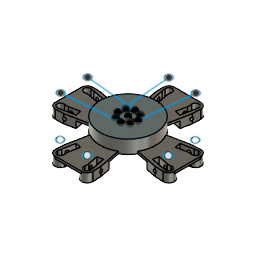
UpperMoulding_v12 (Autodesk Fusion 360 design; units mm, degrees)
Autodesk Fusion 360 part; units mm, degrees
sketch "Sketch3" plane through (0, 0, 0) normal (0, 0, 1) x (1, 0, 0)
  line L0 (-12, 0) -> (12, 0)
  line L1 (0, 0) -> (0, 60) construction
  line L2 (-12, 0) -> (0, 60) construction
  line L3 (0, 60) -> (12, 0) construction
  line L4 (-14.4515, 0.4903) -> (-9.5485, -0.4903)
  line L5 (-14.4515, 0.4903) -> (-9.5485, -0.4903)
  line L6 (-9.5485, -0.4903) -> (-7.5874, 9.3155)
  line L7 (-7.5874, 9.3155) -> (-12.4903, 10.2961)
  line L8 (-12.4903, 10.2961) -> (-14.4515, 0.4903)
  line L9 (-13.4709, 5.3932) -> (-16.4126, 5.9815) construction
  line L10 (-12, -3.0594) -> (12, -3.0594) construction
  circle A0 centre (-12, -3.0594) radius 3
  line L11 (0, 0) -> (0, -3.0594) construction
  line L12 (-14.4515, 0.4903) -> (-14.9594, -2.5678)
  line L13 (-9.5485, -0.4903) -> (-9.0891, -2.3339)
  line L14 (-8.568, 4.4126) -> (-5.6262, 3.8243) construction
  line L15 (-16.1184, 7.4524) -> (-16.7068, 4.5107)
  line L16 (-5.3321, 5.2951) -> (-5.9204, 2.3534)
  line L17 (-16.1184, 7.4524) -> (-13.1767, 6.8641) construction
  line L18 (-16.7068, 4.5107) -> (-13.765, 3.9223) construction
  line L19 (-5.9204, 2.3534) -> (-8.8621, 2.9417) construction
  line L20 (-5.3321, 5.2951) -> (-8.2738, 5.8835) construction
  circle A1 centre (-12, -3.0594) radius 5
  line L21 (-16.7068, 4.5107) -> (-16.9962, -2.8634)
  line L22 (-5.9204, 2.3534) -> (-7.0825, -3.964)
  line L23 (-10.0388, 9.8058) -> (-9.4505, 12.7475)
  line L24 (-16.1184, 7.4524) -> (-14.8437, 13.8262)
  line L25 (-14.8437, 13.8262) -> (-9.4505, 12.7475)
  line L26 (-5.3321, 5.2951) -> (-4.0573, 11.6689)
  line L27 (-4.0573, 11.6689) -> (-9.4505, 12.7475)
  line L28 (9.5485, -0.4903) -> (14.4515, 0.4903)
  line L29 (9.5485, -0.4903) -> (14.4515, 0.4903)
  line L30 (14.4515, 0.4903) -> (12.4903, 10.2961)
  line L31 (12.4903, 10.2961) -> (7.5874, 9.3155)
  line L32 (7.5874, 9.3155) -> (9.5485, -0.4903)
  circle A2 centre (12, -3.0594) radius 3
  line L33 (9.5485, -0.4903) -> (9.0891, -2.3339)
  line L34 (14.4515, 0.4903) -> (14.9594, -2.5678)
  circle A3 centre (12, -3.0594) radius 5
  line L35 (13.4709, 5.3932) -> (16.4126, 5.9815) construction
  line L36 (8.568, 4.4126) -> (5.6262, 3.8243) construction
  line L37 (16.1184, 7.4524) -> (16.7068, 4.5107)
  line L38 (5.3321, 5.2951) -> (5.9204, 2.3534)
  line L39 (5.9204, 2.3534) -> (7.0825, -3.964)
  line L40 (16.7068, 4.5107) -> (16.9962, -2.8634)
  line L41 (10.0388, 9.8058) -> (9.4505, 12.7475) construction
  line L42 (9.4505, 12.7475) -> (14.8437, 13.8262)
  line L43 (14.8437, 13.8262) -> (16.1184, 7.4524)
  line L44 (9.4505, 12.7475) -> (4.0573, 11.6689)
  line L45 (4.0573, 11.6689) -> (5.3321, 5.2951)
  line L46 (-4.0573, 11.6689) -> (4.0573, 11.6689)
  line L47 (-12, -8.0594) -> (12, -8.0594)
  point P0 (0, -3.0594)
  dimension "d11" = 24
  dimension "d12" = 60
  dimension "d13" = 5
  dimension "d14" = 10
  dimension "d15" = 3
  dimension "d16" = 24
  dimension "d17" = 6
  dimension "d18" = 3
  dimension "d19" = 3
  dimension "d20" = 3
  dimension "d21" = 2
  dimension "d22" = 3
  dimension "d23" = 5
  dimension "d24" = 10
  dimension "d25" = 6
  dimension "d26" = 2
  dimension "d27" = 3
  dimension "d28" = 3
  dimension "d29" = 3
  dimension "d30" = 3
  dimension "d31" = 3
  constraint midpoint L0 L1.start
  constraint coincident L1.start L11.start
  constraint horizontal L0
  constraint vertical L1
  constraint midpoint L0.start L4
  constraint perpendicular L2 L4
  constraint perpendicular L5 L6
  constraint parallel L5 L7
  constraint parallel L6 L8
  constraint midpoint L8 L9.start
  constraint perpendicular L8 L9
  constraint midpoint L10 P0
  constraint perpendicular L1 L10
  constraint coincident L10.start A0.centre
  constraint coincident P0 L11.end
  constraint perpendicular L10 L11
  constraint tangent L5 A0
  constraint coincident A0 L12.end
  constraint tangent A0 L12
  constraint coincident A0 L13.end
  constraint tangent A0 L13
  constraint midpoint L6 L14.start
  constraint perpendicular L6 L14
  constraint midpoint L9.end L15
  constraint perpendicular L9 L15
  constraint midpoint L14.end L16
  constraint perpendicular L14 L16
  constraint coincident L8 L17.end
  constraint perpendicular L8 L17
  constraint coincident L8 L18.end
  constraint perpendicular L8 L18
  constraint coincident L6 L19.end
  constraint perpendicular L6 L19
  constraint coincident L6 L20.end
  constraint perpendicular L6 L20
  constraint concentric A0 A1
  constraint coincident A1 L21.end
  constraint tangent A1 L21
  constraint coincident A1 L22.end
  constraint tangent A1 L22
  constraint midpoint L7 L23.start
  constraint perpendicular L7 L23
  constraint perpendicular L17 L24
  constraint perpendicular L20 L26
  constraint perpendicular L24 L25
  constraint perpendicular L26 L27
  constraint midpoint L0.end L28
  constraint perpendicular L3 L28
  constraint perpendicular L29 L30
  constraint parallel L29 L31
  constraint parallel L30 L32
  constraint coincident L10.end A2.centre
  constraint coincident A2 L33.end
  constraint tangent A2 L33
  constraint coincident A2 L34.end
  constraint tangent A2 L34
  constraint concentric A2 A3
  constraint midpoint L30 L35.start
  constraint perpendicular L30 L35
  constraint midpoint L32 L36.start
  constraint perpendicular L32 L36
  constraint midpoint L35.end L37
  constraint perpendicular L35 L37
  constraint midpoint L36.end L38
  constraint perpendicular L36 L38
  constraint coincident A3 L39.end
  constraint tangent A3 L39
  constraint coincident A3 L40.end
  constraint tangent A3 L40
  constraint midpoint L31 L41.start
  constraint perpendicular L31 L41
  constraint perpendicular L41 L42
  constraint perpendicular L41 L44
  constraint perpendicular L44 L45
  constraint perpendicular L42 L43
  constraint coincident A1 L47.start
  constraint coincident A3 L47.end
  constraint tangent A1 L47
  constraint tangent A3 L47
  measures "d11" distance of L0.start L0.end
  measures "d12" distance of L1.start L1.end
  measures "d13" distance of L4.start L4.end
  measures "d14" distance of L4.start L7.end
  measures "d15" distance of L9.start L9.end
  measures "d16" distance of L10.start L10.end
  measures "d17" diameter of A0
  measures "d18" distance of L14.start L14.end
  measures "d19" distance of L15.start L15.end
  measures "d20" distance of L16.start L16.end
  measures "d21" distance of A0 A1
  measures "d22" distance of L23.start L23.end
  measures "d23" distance of L28.start L28.end
  measures "d24" distance of L28.start L31.end
  measures "d25" diameter of A2
  measures "d26" distance of A2 A3
  measures "d27" distance of L35.start L35.end
  measures "d28" distance of L36.start L36.end
  measures "d29" distance of L37.start L37.end
  measures "d30" distance of L38.start L38.end
  measures "d31" distance of L41.start L41.end
extrude "Extrude4" add sketch "Sketch3" along normal blind 8 contours L0 L6 A1 | L0 L6 L8 A0 L12 L13 A1 | L0 L6 L7 L16 A1 L22 L23 L26 L27 | L0 A1 L22 | L7 L8 L15 A1 L21 L23 L24 L25 | L0 L30 L31 L32 A3 L37 L38 L39 L40 L42 L43 L44 L45 | L0 A3 L39 | L0 L32 A3 | L0 L30 L32 A2 L33 L34 A3 makes body 1 at (-10.4638, 11.9304, 0) makes body 2 at (10.4638, 11.9304, 0)
sketch "Sketch4" plane through (-16.9317, 3.3863, 0) normal (-0.980581, 0.196116, 0) x (-0.196116, -0.980581, 0)
  line L0 (-10.6466, 0) -> (-1.1466, 0)
  line L1 (-1.1466, 0) -> (-1.1466, 8)
  line L2 (-1.1466, 8) -> (-10.6466, 8)
  line L3 (-10.6466, 8) -> (-10.6466, 0)
  line L4 (-1.1466, 4) -> (-1.6466, 4) construction
  circle A0 centre (-1.6466, 4) radius 1.5
  dimension "d34" = 3
  dimension "d41" = 0.5
  constraint midpoint L1 L4.start
  constraint perpendicular L1 L4
  constraint coincident L4.end A0.centre
  measures "d34" diameter of A0
  measures "d41" distance of L4.start L4.end
extrude "Extrude5" cut sketch "Sketch4" against normal blind 10 contours L1 A0 | L1 A0 bodies 1
sketch "Sketch5" plane through (16.9317, 3.3863, 0) normal (0.980581, 0.196116, 0) x (-0.196116, 0.980581, 0)
  line L0 (1.1466, 0) -> (10.6466, 0)
  line L1 (10.6466, 0) -> (10.6466, 8)
  line L2 (10.6466, 8) -> (1.1466, 8)
  line L3 (1.1466, 8) -> (1.1466, 0)
  line L4 (1.1466, 4) -> (1.6466, 4) construction
  circle A0 centre (1.6466, 4) radius 1.5
  dimension "d37" = 0.5
  dimension "d38" = 3
  constraint midpoint L3 L4.start
  constraint perpendicular L3 L4
  constraint coincident L4.end A0.centre
  measures "d37" distance of L4.start L4.end
  measures "d38" diameter of A0
extrude "Extrude6" cut sketch "Sketch5" against normal blind 10 contours L3 A0 | L3 A0 bodies 2
move_face "OffsetFaces1" offset -1 2 faces at (-9.2217, 9.6424, 5.3333) (10.856, 9.9692, 2.6667) on bodies 1 2
extrude "Extrude7" add sketch "Sketch3" along normal blind 2 from surface at 6 contours L0 L16 L22 L26 L38 L39 L45 L46 | L0 A1 L22 A3 L39 L47 bodies 1 2
sketch "Sketch6" plane through (0, 0, 8) normal (0, 0, 1) x (-1, 0, 0)
  line L0 (-7.3913, -10.2961) -> (-12.2942, -11.2767)
  line L1 (-12.2942, -11.2767) -> (-14.4515, -0.4903)
  line L2 (-14.4515, -0.4903) -> (-14.9594, 2.5678)
  arc A0 (-9.0891, 2.3339) -> (-14.9594, 2.5678) centre (-12, 3.0594) ccw
  line L3 (-9.0891, 2.3339) -> (-9.5485, 0.4903)
  line L4 (-9.5485, 0.4903) -> (-7.3913, -10.2961)
  line L5 (12.2942, -11.2767) -> (7.3913, -10.2961)
  line L6 (7.3913, -10.2961) -> (9.5485, 0.4903)
  line L7 (9.5485, 0.4903) -> (9.0891, 2.3339)
  arc A1 (14.9594, 2.5678) -> (9.0891, 2.3339) centre (12, 3.0594) ccw
  line L8 (14.9594, 2.5678) -> (14.4515, -0.4903)
  line L9 (14.4515, -0.4903) -> (12.2942, -11.2767)
  line L10 (4.0573, -11.6689) -> (14.8437, -13.8262)
  line L11 (14.8437, -13.8262) -> (16.7068, -4.5107)
  line L12 (16.7068, -4.5107) -> (16.9962, 2.8634)
  arc A2 (16.9962, 2.8634) -> (12, 8.0594) centre (12, 3.0594) ccw
  line L13 (12, 8.0594) -> (-12, 8.0594)
  arc A3 (-12, 8.0594) -> (-16.9962, 2.8634) centre (-12, 3.0594) ccw
  line L14 (-16.9962, 2.8634) -> (-16.7068, -4.5107)
  line L15 (-16.7068, -4.5107) -> (-14.8437, -13.8262)
  line L16 (-14.8437, -13.8262) -> (-4.0573, -11.6689)
  line L17 (-4.0573, -11.6689) -> (4.0573, -11.6689)
  line L18 (-12, 3.0594) -> (0, -45.6677)
  line L19 (0, -45.6677) -> (12, 3.0594)
  circle A4 centre (0, -45.6677) radius 60
  circle A5 centre (0, -45.6677) radius 25
  line L20 (14.8437, -13.8262) -> (12.7735, -24.1773)
  line L21 (-14.8437, -13.8262) -> (-12.7735, -24.1773)
  dimension "d48" = 50.183
  dimension "d49" = 50.183
  dimension "d50" = 120
  dimension "d53" = 50
  constraint coincident A0.centre A3.centre
  constraint coincident A1.centre A2.centre
  constraint coincident L18.end L19.start
  constraint concentric A4 A5
  constraint coincident L10.end L11.start
  constraint coincident A5 L20.end
  constraint perpendicular L10 L20
  constraint coincident L15.end L16.start
  constraint perpendicular L16 L21
  measures "d48" distance of A0.centre L18.end
  measures "d49" distance of L18.end A1.centre
  measures "d50" diameter of A4
  measures "d53" diameter of A5
extrude "Extrude8" add sketch "Sketch6" against normal blind 2 contours L10 L16 L17 L18 L19 A5 | L10 L19 A5 L20 | L18 L19 A5 | L18 L19 A5 | L16 L18 A5 L21 bodies 1
fillet "Fillet2" radius 8 2 edges at (-9.5485, -0.4903, 4) (9.5485, -0.4903, 4) on bodies 1
pattern_circular "C-Pattern1" count 4 over 360 about axis through (0, 45.6677, 8) along (0, 0, 1) of bodies 1 makes body 3 at (40.2418, 60.1519, 0) makes body 4 at (-14.4841, 85.9096, 0) makes body 5 at (-40.2418, 31.1836, 0)
combine "Combine1" operation add target body 5 tool bodies 4 1 3
sketch "Sketch7" plane through (0, 0, 8) normal (0, 0, 1) x (-1, 0, 0)
  arc A0 (-44.397, -36.4714) -> (-47.9006, -36.5535) centre (-45.9659, -44.316) ccw
  line L0 (-47.9006, -36.5535) -> (-48.0016, -36.5787)
  arc A1 (-48.2355, -30.7083) -> (-48.0016, -36.5787) centre (-48.7271, -33.6677) ccw
  line L1 (-48.2355, -30.7083) -> (-45.1774, -31.2163)
  line L2 (-45.1774, -31.2163) -> (-34.391, -33.3735)
  line L3 (-34.391, -33.3735) -> (-35.3716, -38.2765)
  line L4 (-35.3716, -38.2765) -> (-44.397, -36.4714)
  arc A2 (-47.9006, -54.7819) -> (-44.397, -54.8641) centre (-45.9659, -47.0194) ccw
  line L5 (-44.397, -54.8641) -> (-35.3716, -53.059)
  line L6 (-35.3716, -53.059) -> (-34.391, -57.9619)
  line L7 (-34.391, -57.9619) -> (-45.1774, -60.1192)
  line L8 (-45.1774, -60.1192) -> (-48.2355, -60.6272)
  arc A3 (-48.0016, -54.7568) -> (-48.2355, -60.6272) centre (-48.7271, -57.6677) ccw
  line L9 (-48.0016, -54.7568) -> (-47.9006, -54.7819)
  arc A4 (-9.1142, 2.2329) -> (-9.1963, -1.2708) centre (-1.3517, 0.2982) ccw
  line L10 (-9.1963, -1.2708) -> (-7.3913, -10.2961)
  line L11 (-7.3913, -10.2961) -> (-12.2942, -11.2767)
  line L12 (-12.2942, -11.2767) -> (-14.4515, -0.4903)
  line L13 (-14.4515, -0.4903) -> (-14.9594, 2.5678)
  arc A5 (-9.0891, 2.3339) -> (-14.9594, 2.5678) centre (-12, 3.0594) ccw
  line L14 (-9.0891, 2.3339) -> (-9.1142, 2.2329)
  arc A6 (9.1963, -1.2708) -> (9.1142, 2.2329) centre (1.3517, 0.2982) ccw
  line L15 (9.1142, 2.2329) -> (9.0891, 2.3339)
  arc A7 (14.9594, 2.5678) -> (9.0891, 2.3339) centre (12, 3.0594) ccw
  line L16 (14.9594, 2.5678) -> (14.4515, -0.4903)
  line L17 (14.4515, -0.4903) -> (12.2942, -11.2767)
  line L18 (12.2942, -11.2767) -> (7.3913, -10.2961)
  line L19 (7.3913, -10.2961) -> (9.1963, -1.2708)
  arc A8 (9.1142, -93.5683) -> (9.1963, -90.0647) centre (1.3517, -91.6336) ccw
  line L20 (9.1963, -90.0647) -> (7.3913, -81.0393)
  line L21 (7.3913, -81.0393) -> (12.2942, -80.0588)
  line L22 (12.2942, -80.0588) -> (14.4515, -90.8452)
  line L23 (14.4515, -90.8452) -> (14.9594, -93.9032)
  arc A9 (9.0891, -93.6693) -> (14.9594, -93.9032) centre (12, -94.3949) ccw
  line L24 (9.0891, -93.6693) -> (9.1142, -93.5683)
  arc A10 (-9.1963, -90.0647) -> (-9.1142, -93.5683) centre (-1.3517, -91.6336) ccw
  line L25 (-9.1142, -93.5683) -> (-9.0891, -93.6693)
  arc A11 (-14.9594, -93.9032) -> (-9.0891, -93.6693) centre (-12, -94.3949) ccw
  line L26 (-14.9594, -93.9032) -> (-14.4515, -90.8452)
  line L27 (-14.4515, -90.8452) -> (-12.2942, -80.0588)
  line L28 (-12.2942, -80.0588) -> (-7.3913, -81.0393)
  line L29 (-7.3913, -81.0393) -> (-9.1963, -90.0647)
  line L30 (21.4904, -58.4412) -> (41.1571, -62.3745)
  line L31 (41.1571, -62.3745) -> (48.5311, -62.6639)
  arc A12 (48.5311, -62.6639) -> (53.7271, -57.6677) centre (48.7271, -57.6677) ccw
  line L32 (53.7271, -57.6677) -> (53.7271, -33.6677)
  arc A13 (53.7271, -33.6677) -> (48.5311, -28.6716) centre (48.7271, -33.6677) ccw
  line L33 (48.5311, -28.6716) -> (41.1571, -28.9609)
  line L34 (41.1571, -28.9609) -> (21.4904, -32.8943)
  arc A14 (21.4904, -32.8943) -> (12.7735, -24.1773) centre (0, -45.6677) ccw
  line L35 (12.7735, -24.1773) -> (16.7068, -4.5107)
  line L36 (16.7068, -4.5107) -> (16.9962, 2.8634)
  arc A15 (16.9962, 2.8634) -> (12, 8.0594) centre (12, 3.0594) ccw
  line L37 (12, 8.0594) -> (-12, 8.0594)
  arc A16 (-12, 8.0594) -> (-16.9962, 2.8634) centre (-12, 3.0594) ccw
  line L38 (-16.9962, 2.8634) -> (-16.7068, -4.5107)
  line L39 (-16.7068, -4.5107) -> (-12.7735, -24.1773)
  arc A17 (-12.7735, -24.1773) -> (-21.4904, -32.8943) centre (0, -45.6677) ccw
  line L40 (-21.4904, -32.8943) -> (-41.1571, -28.9609)
  line L41 (-41.1571, -28.9609) -> (-48.5311, -28.6716)
  arc A18 (-48.5311, -28.6716) -> (-53.7271, -33.6677) centre (-48.7271, -33.6677) ccw
  line L42 (-53.7271, -33.6677) -> (-53.7271, -57.6677)
  arc A19 (-53.7271, -57.6677) -> (-48.5311, -62.6639) centre (-48.7271, -57.6677) ccw
  line L43 (-48.5311, -62.6639) -> (-41.1571, -62.3745)
  line L44 (-41.1571, -62.3745) -> (-21.4904, -58.4412)
  arc A20 (-21.4904, -58.4412) -> (-12.7735, -67.1582) centre (0, -45.6677) ccw
  line L45 (-12.7735, -67.1582) -> (-16.7068, -86.8248)
  line L46 (-16.7068, -86.8248) -> (-16.9962, -94.1988)
  arc A21 (-16.9962, -94.1988) -> (-12, -99.3949) centre (-12, -94.3949) ccw
  line L47 (-12, -99.3949) -> (12, -99.3949)
  arc A22 (12, -99.3949) -> (16.9962, -94.1988) centre (12, -94.3949) ccw
  line L48 (16.9962, -94.1988) -> (16.7068, -86.8248)
  line L49 (16.7068, -86.8248) -> (12.7735, -67.1582)
  arc A23 (12.7735, -67.1582) -> (21.4904, -58.4412) centre (0, -45.6677) ccw
  arc A24 (44.397, -54.8641) -> (47.9006, -54.7819) centre (45.9659, -47.0194) ccw
  line L50 (47.9006, -54.7819) -> (48.0016, -54.7568)
  arc A25 (48.2355, -60.6272) -> (48.0016, -54.7568) centre (48.7271, -57.6677) ccw
  line L51 (48.2355, -60.6272) -> (45.1774, -60.1192)
  line L52 (45.1774, -60.1192) -> (34.391, -57.9619)
  line L53 (34.391, -57.9619) -> (35.3716, -53.059)
  line L54 (35.3716, -53.059) -> (44.397, -54.8641)
  arc A26 (47.9006, -36.5535) -> (44.397, -36.4714) centre (45.9659, -44.316) ccw
  line L55 (44.397, -36.4714) -> (35.3716, -38.2765)
  line L56 (35.3716, -38.2765) -> (34.391, -33.3735)
  line L57 (34.391, -33.3735) -> (45.1774, -31.2163)
  line L58 (45.1774, -31.2163) -> (48.2355, -30.7083)
  arc A27 (48.0016, -36.5787) -> (48.2355, -30.7083) centre (48.7271, -33.6677) ccw
  line L59 (48.0016, -36.5787) -> (47.9006, -36.5535)
  circle A28 centre (0, -45.6677) radius 25
  constraint concentric A14 A28
extrude "Extrude9" add sketch "Sketch7" along normal blind 10 contours A14 A17 A20 A23 A28 bodies 5
sketch "Sketch8" plane through (0, 0, 18) normal (0, 0, 1) x (-1, 0, 0)
  circle A0 centre (0, -45.6677) radius 25
  circle A1 centre (0, -45.6677) radius 6
  line L0 (0, -45.6677) -> (1.3892, -53.5462) construction
  circle A2 centre (1.3892, -53.5462) radius 1
  circle A3 centre (6.5532, -50.2563) radius 1
  circle A4 centre (7.8785, -44.2785) radius 1
  circle A5 centre (4.5886, -39.1145) radius 1
  circle A6 centre (-1.3892, -37.7893) radius 1
  circle A7 centre (-6.5532, -41.0791) radius 1
  circle A8 centre (-7.8785, -47.0569) radius 1
  circle A9 centre (-4.5886, -52.2209) radius 1
  line L1 (0, -45.6677) -> (-6, -45.6677)
  circle A10 centre (-12.3401, -94.276) radius 3
  circle A11 centre (11.9412, -94.2971) radius 3
  circle A12 centre (48.6083, -58.0078) radius 3
  circle A13 centre (48.6294, -33.7265) radius 3
  circle A14 centre (12.3401, 2.9406) radius 3
  circle A15 centre (-11.9412, 2.9617) radius 3
  circle A16 centre (-48.6083, -33.3277) radius 3
  circle A17 centre (-48.6294, -57.609) radius 3
  line L2 (-12.3401, -94.276) -> (-7.8785, -47.0569)
  line L3 (7.8785, -44.2785) -> (11.9412, -94.2971)
  line L4 (1.3892, -53.5462) -> (48.6083, -58.0078)
  line L5 (-1.3892, -37.7893) -> (48.6294, -33.7265)
  dimension "d60" = 12
  dimension "d61" = 8
  dimension "d62" = 2
  dimension "d64" = 360
  dimension "d65" = 100
  dimension "d66" = 6
  dimension "d67" = 6
  dimension "d69" = 360
  constraint concentric A0 A1
  constraint coincident A0.centre A1.centre
  constraint coincident L0.end A2.centre
  constraint coincident A1 L1.end
  constraint horizontal L1
  constraint coincident A10.centre L2.start
  constraint coincident A8.centre L2.end
  constraint coincident A4.centre L3.start
  constraint coincident A11.centre L3.end
  constraint coincident A12.centre L4.end
  constraint coincident A6.centre L5.start
  constraint coincident A13.centre L5.end
  measures "d60" diameter of A1
  measures "d61" distance of A0.centre L0.end
  measures "d62" diameter of A2
  measures "d65" angle of L0 L1
  measures "d66" diameter of A10
  measures "d67" diameter of A11
